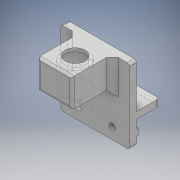
# Autodesk Inventor part: Estrutura - Suporte Rolamento Z Motor
Saved by Autodesk Inventor 2017 (Build 210142000, 142)
## iProperties
Created: 2020-08-03
Part Number: Estrutura - Suporte Rolamento Z Motor
Material: Generic
Document SubType Name: Modeling
Designer: ale
Density: 1 g/cm^3
Appearance: Default
Author: ale
Autodesk Inventor part; units mm, degrees
ref_plane "YZ Plane" through (0, 0, 0) normal (1, 0, 0) x (0, 1, 0)
ref_plane "XZ Plane" through (0, 0, 0) normal (0, 1, 0) x (-1, 0, 0)
ref_plane "XY Plane" through (0, 0, 0) normal (0, 0, 1) x (1, 0, 0)
sketch "Sketch1" plane through (0, 0, 0) normal (0, 0, 1) x (1, 0, 0)
  circle A0 centre (0, 0) radius 11.4
  line L0 (-15, 17.5) -> (15, 17.5)
  line L1 (15, 17.5) -> (15, -17.5)
  line L2 (15, -17.5) -> (-15, -17.5)
  line L3 (-15, -17.5) -> (-15, 17.5)
  line L4 (-15, 17.5) -> (15, -17.5) construction
  line L5 (15, 17.5) -> (-15, -17.5) construction
  dimension "d0" = 22.8
  dimension "d1" = 30
  dimension "d2" = 35
  constraints: 12 end point, 2 midpoint, 2 parallel, 1 centre point, 1 coincident, 1 horizontal, 1 perpendicular
  measures "d0" diameter of A0
  measures "d1" distance of L1.end L2.end
  measures "d2" distance of L0.end L1.end
extrude "Extrusion1" add sketch "Sketch1" along normal blind 25
sketch "Sketch3" plane through (-15, 17.5, 0) normal (0, 1, 0) x (1, 0, 0)
  line L0 (30, 0) -> (0, 0) projected
  line L1 (0, 0) -> (30, -25)
  line L2 (45, 40) -> (-15, 40)
  line L3 (-15, 40) -> (-15, -25)
  line L4 (-15, -25) -> (45, -25)
  line L5 (45, -25) -> (45, 40)
  line L6 (0, 0) -> (30, 0) projected
  line L7 (30, 0) -> (45, 0)
  line L8 (30, -25) -> (0, -25) projected
  point P0 (15, 0)
  point P1 (15, -12.5)
  dimension "d8" = 60
  dimension "d9" = 65
  dimension "d27" = 0
  constraints: 12 end point, 2 parallel, 1 horizontal, 1 midpoint, 1 perpendicular, 1 point on line
  measures "d8" distance of L4.end L3.end
  measures "d9" distance of L3.end L2.end
  measures "d27" distance between parallel lines of L4 L8
extrude "Extrusion3" add sketch "Sketch3" along normal blind 6
sketch "Sketch4" plane through (-15, 23.5, 0) normal (0, 1, 0) x (1, 0, 0)
  line L0 (-15, 33) -> (45, 33)
  line L1 (-15, 27) -> (45, 27)
  line L2 (45, 33) -> (45, 27)
  line L3 (-15, 27) -> (-15, 33)
  line L4 (45, 40) -> (-15, 40) projected
  dimension "d20" = 7
  dimension "d21" = 13
  constraints: 8 end point, 1 perpendicular
  measures "d20" distance from line of L4.start L0
  measures "d21" distance between parallel lines of L4 L1
sketch "Sketch5" plane through (0, 0, 25) normal (0, 0, 1) x (1, 0, 0)
  circle A0 centre (0, 0) radius 11.4
  circle A1 centre (0, 0) radius 8.5
  dimension "d24" = 17
  constraints: 2 centre point, 2 coincident
  measures "d24" diameter of A1
extrude "Extrusion5" add sketch "Sketch5" against normal blind 3
chamfer "Chamfer1" distance 5 angle 45 3 edges at (15, 17.5, 12.5) (-15, 17.5, 12.5) (0, 17.5, 0)
extrude "Extrusion6" add sketch "Sketch4" along normal blind 1.5
sketch "Sketch8" plane through (-15, 23.5, 0) normal (0, 1, 0) x (1, 0, 0)
  line L0 (45, 40) -> (-15, 40) projected
  line L1 (-15, 20) -> (45, 20)
  line L2 (45, 20) -> (45, 14)
  line L3 (45, 14) -> (-15, 14)
  line L4 (-15, 14) -> (-15, 20)
  point P0 (43, 40)
  point P1 (-13, 40)
  point P2 (15, 11.0426)
  dimension "d47" = 6
  dimension "d50" = 20
  constraints: 8 end point, 2 parallel, 1 horizontal, 1 perpendicular
  measures "d47" distance of L1.end L2.end
  measures "d50" distance between parallel lines of L1 L0
extrude "Extrusion7" add sketch "Sketch8" along normal blind 20
sketch "Sketch10" plane through (-15, 25, 0) normal (0, 1, 0) x (1, 0, 0)
  line L0 (45, 33) -> (-15, 33) projected
  line L1 (15, 33) -> (15, 27)
  line L2 (45, 27) -> (-15, 27) projected
  line L3 (0, 33) -> (0, 27)
  line L4 (30, 33) -> (30, 27)
  point P0 (15, 0)
  point P1 (0, 30)
  point P2 (30, 30)
  dimension "d51" = 15
  dimension "d52" = 15
  constraints: 6 end point, 4 midpoint, 2 parallel
  measures "d51" distance between parallel lines of L1 L3
  measures "d52" distance between parallel lines of L1 L4
hole "Hole2" at (-15, 25, -30) at (15, 25, -30) direction (0, -1, 0) diameter 5.5 end through all counterbore diameter 10 counterbore depth 1.5
sketch "Sketch11" plane through (30, 23.5, -20) normal (0, 0, -1) x (-1, 0, 0)
  line L0 (60, 0) -> (60, 20) projected
  line L1 (60, 10) -> (0, 10)
  line L2 (0, 0) -> (0, 20) projected
  line L3 (60, 20) -> (0, 20) projected
  line L4 (30, 20) -> (30, 10)
  point P0 (30, -23.5)
  constraints: 4 end point, 4 midpoint, 1 coincident
hole "Hole3" at (0, 33.5, -20) direction (0, 0, 1) diameter 5.5 end through all
fillet "Fillet2" radius 2 10 edges at (-30, 20.5, -40) (30, 20.5, -40) (-30, 20.5, 25) (30, 20.5, 25) (30, 43.5, -17) (-30, 43.5, -17) (-15, -17.5, 12.5) (15, -17.5, 12.5) (0, -17.5, 25) (0, -17.5, 0)
body "Solid1"
